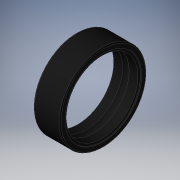
# Autodesk Inventor part: 6000DDU Outer ring
Saved by Autodesk Inventor 2023 (Build 270158000, 158)
## iProperties
Created: 2023-07-21
Part Number: 6000DDU Outer ring
Material: Generic
Catalog Web Link: www.cadenas.de
Description: contact_sealed_type_dd_ddu_OR-NSK
Vendor: NSK_RB
Document SubType Name: Modeling
Designer: psAdmin
Manufacturer: NSK_RB
Mass: 1.27901 g
Surface Area: 15.1976 cm^2
Volume: 1.27901 cm^3
Density: 1 g/cm^3
Appearance: PSOLRGB-128-128-128
Category: PARTsolutions
Company: NSK_RB
PSOL_IDENT_0: {$CADENAS_DATA/23d-libs/nsk_rb/roller_bearings/deep_groove_bb/single_row_dgbb/contact_sealed_type_dd
PSOL_IDENT_1: _ddu_1_or.prj},199 {VTYP=3D},{NB=6000DDU Outer ring},{LINA=6000DDU Outer ring},{NN=contact_sealed_ty
PSOL_IDENT_2: pe_dd_ddu_OR},{DATE=15.09.2022 00:32:48},{GEOMDATE=08.08.2022 08:01:00},{VERSION=},{LINEID=30},{WBVA
PSOL_IDENT_3: R=},{WBNUMERIC=}  {NB=6000DDU Outer ring},{LINA=6000DDU Outer ring},{KT=DUMMY},{IDNR=},{STAN=Standar
PSOL_IDENT_4: d},{ORDER=6000DDU},{SD=10},{X=10},{DI1=14.57},{DI2=13.2},{SDE1=21.50},{SDE2=23.00},{D=26},{DD=26},{B=
PSOL_IDENT_5: 8},{R=0.3},{CR1=4550},{COR1=1970},{CR2=465},{COR2=201},{FO=12.4},{LG=22000},{A=1.35},{BB=0.87},{DD1=
PSOL_IDENT_6: 24.50},{RO=0.20},{RN=0.3},{DD2=28.7},{F=0.84},{DAM1=12.0},{DA1=13.0},{DA2=24.0},{RA=0.3},{DX=29.4},{
PSOL_IDENT_7: CY=1.9},{MASS=0.018},{SC=1},{DIST=1.133}
NB: 6000DDU Outer ring
NN: contact_sealed_type_dd_ddu_OR
NT: NSK
NBSYN: $ORDER. Outer ring
LINA: 6000DDU Outer ring
CATALOG: NSK Rolling Bearing
STAN: Standard
ORDER: 6000DDU
SD: 10
X: 10
DI1: 14.57
DI2: 13.2
SDE1: 21.5
SDE2: 23
D: 26
DD: 26
B: 8
R: 0.3
CR1: 4550
COR1: 1970
CR2: 465
COR2: 201
FO: 12.4
LG: 22000
A: 1.35
BB: 0.87
DD1: 24.5
RO: 0.2
RN: 0.3
DD2: 28.7
F: 0.84
DAM1: 12
DA1: 13
DA2: 24
RA: 0.3
DX: 29.4
CY: 1.9
MASS: 0.018
SC: 1
SUPPLIER: NSK_RB
ARTICLENO: 6000DDU Outer ring
BOMINFO: 6000DDU Outer ring
CREATOR: CADENAS GmbH
Title: 6000DDU Outer ring
Author: Cadenas PARTsolutions
Comments: NSK
Autodesk Inventor part; units mm, degrees
sketch "Sketch_1" plane through (0, 0, 0) normal (0, 0, 1) x (1, 0, 0)
  line L0 (8, 0) -> (0, 0)
  line L1 (0, 11.5) -> (0.368, 11.5)
  line L2 (0.368, 11.5) -> (0.368, 10.75)
  line L3 (0.368, 10.75) -> (3.0318, 10.75)
  arc A0 (4.9682, 10.75) -> (3.0318, 10.75) centre (4, 9) ccw
  line L4 (4.9682, 10.75) -> (7.632, 10.75)
  line L5 (7.632, 10.75) -> (7.632, 11.5)
  line L6 (7.632, 11.5) -> (8, 11.5)
  line L7 (8, 11.5) -> (8, 12.7)
  arc A1 (8, 12.7) -> (7.7, 13) centre (7.7, 12.7) ccw
  line L8 (7.7, 13) -> (0.3, 13)
  arc A2 (0.3, 13) -> (0, 12.7) centre (0.3, 12.7) ccw
  line L9 (0, 12.7) -> (0, 11.5)
  constraints: 20 end point, 6 point on circle, 3 centre point
revolve "Revolution1" add sketch "Sketch_1" angle 360 about axis through (8, 0, 0) along (1, 0, 0)
ref_plane "ip_cst_1_or_1_XY" through (0, 0, 0) normal (1, 0, 0) x (0, 0, -1)
ref_plane "ip_cst_1_or_1_YZ" through (0, 0, 0) normal (0, 0, -1) x (0, 1, 0)
ref_plane "ip_cst_1_or_1_ZX" through (0, 0, 0) normal (0, 1, 0) x (1, 0, 0)
ref_plane "ip_cst_1_or_2_XY" through (0, 0, 0) normal (-1, 0, 0) x (0, 0, -1)
ref_plane "ip_cst_1_or_2_YZ" through (0, 0, 0) normal (0, 0, -1) x (0, -1, 0)
ref_plane "ip_cst_1_or_2_ZX" through (0, 0, 0) normal (0, -1, 0) x (-1, 0, 0)
ref_plane "ip_cst_1_or_3_XY" through (0.368, 0, 0) normal (1, 0, 0) x (0, 0, -1)
ref_plane "ip_cst_1_or_3_YZ" through (0.368, 0, 0) normal (0, 0, -1) x (0, 1, 0)
ref_plane "ip_cst_1_or_3_ZX" through (0.368, 0, 0) normal (0, 1, 0) x (1, 0, 0)
ref_plane "ip_cst_1_or_4_XY" through (7.632, 0, 0) normal (-1, 0, 0) x (0, 0, -1)
ref_plane "ip_cst_1_or_4_YZ" through (7.632, 0, 0) normal (0, 0, -1) x (0, -1, 0)
ref_plane "ip_cst_1_or_4_ZX" through (7.632, 0, 0) normal (0, -1, 0) x (-1, 0, 0)
body "Solid1"
